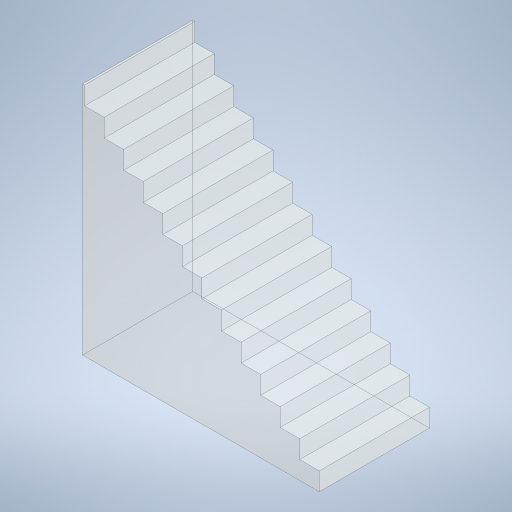
# Autodesk Inventor part: Stairs_Between_Basement_And_First_Floor
Saved by Autodesk Inventor 2024 (Build 280153000, 153)
## iProperties
Created: 2023-05-16
Part Number: Stairs_Between_Basement_And_First_Floor
Material: Steel
Document SubType Name: Modeling
Designer: Tom
Density: 7.85 g/cm^3
Appearance: Clear
Mass: 2.17052e+07 g
Surface Area: 147038 cm^2
Volume: 2.765e+06 cm^3
Author: Tom
Autodesk Inventor part; units mm, degrees
ref_plane "YZ Plane" through (0, 0, 0) normal (1, 0, 0) x (0, 1, 0)
ref_plane "XZ Plane" through (0, 0, 0) normal (0, 1, 0) x (-1, 0, 0)
ref_plane "XY Plane" through (0, 0, 0) normal (0, 0, 1) x (1, 0, 0)
sketch "Sketch1" plane through (0, 0, 0) normal (0, 0, 1) x (1, 0, 0)
  line L0 (-182.5625, 168.5192) -> (-182.5625, 337.0385)
  line L1 (-182.5625, 337.0385) -> (-365.125, 337.0385)
  line L2 (-365.125, 337.0385) -> (-365.125, 505.5577)
  line L3 (-365.125, 505.5577) -> (-547.6875, 505.5577)
  line L4 (-547.6875, 505.5577) -> (-547.6875, 674.0769)
  line L5 (-547.6875, 674.0769) -> (-730.25, 674.0769)
  line L6 (-730.25, 674.0769) -> (-730.25, 842.5962)
  line L7 (-730.25, 842.5962) -> (-912.8125, 842.5962)
  line L8 (-912.8125, 842.5962) -> (-912.8125, 1011.1154)
  line L9 (-912.8125, 1011.1154) -> (-1095.375, 1011.1154)
  line L10 (-1095.375, 1011.1154) -> (-1095.375, 1179.6346)
  line L11 (-1095.375, 1179.6346) -> (-1277.9375, 1179.6346)
  line L12 (-1277.9375, 1179.6346) -> (-1277.9375, 1348.1538)
  line L13 (-1277.9375, 1348.1538) -> (-1460.5, 1348.1538)
  line L14 (-1460.5, 1348.1538) -> (-1460.5, 1516.6731)
  line L15 (-1460.5, 1516.6731) -> (-1643.0625, 1516.6731)
  line L16 (-1643.0625, 1516.6731) -> (-1643.0625, 1685.1923)
  line L17 (-1643.0625, 1685.1923) -> (-1825.625, 1685.1923)
  line L18 (-1825.625, 1685.1923) -> (-1825.625, 1853.7115)
  line L19 (-1825.625, 1853.7115) -> (-2008.1875, 1853.7115)
  line L20 (-2008.1875, 1853.7115) -> (-2008.1875, 2022.2308)
  line L21 (-2008.1875, 2022.2308) -> (-2190.75, 2022.2308)
  line L22 (-2190.75, 2022.2308) -> (-2190.75, 2190.75)
  line L23 (-2190.75, 2190.75) -> (-2209.8, 2190.75)
  line L24 (-2209.8, 2190.75) -> (-2209.8, 0)
  line L25 (-182.5625, 168.5192) -> (0, 168.5192)
  line L26 (0, 168.5192) -> (0, 0)
  line L27 (0, 0) -> (-2209.8, 0)
  point P0 (-2590.1533, 586.4349)
  dimension "d3" = 19.05
  dimension "d9" = 2190.75
  dimension "d12" = 2209.8
  constraints: 56 end point, 24 perpendicular, 23 parallel, 3 horizontal, 1 coincident, 1 vertical
  measures "d3" distance between parallel lines of L24 L22
  measures "d9" distance of L23.end L24.end
  measures "d12" distance between parallel lines of L26 L24
extrude "Extrusion1" add sketch "Sketch1" along normal blind 1028.7
body "Solid1"
